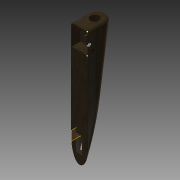
# Autodesk Inventor part: Version 1
Saved by Autodesk Inventor 2015 SP2 (Build 190223200, 223)
## iProperties
Created: 2016-03-30
Part Number: Version 1
Material: Wood (Maple)
Document SubType Name: Modeling
Designer: cvhssub1
Density: 0.67 g/cm^3
Appearance: Natural Maple - Glossy Dark Tint
Author: cvhssub1
Autodesk Inventor part; units mm, degrees
ref_plane "YZ Plane" through (0, 0, 0) normal (1, 0, 0) x (0, 1, 0)
ref_plane "XZ Plane" through (0, 0, 0) normal (0, 1, 0) x (-1, 0, 0)
ref_plane "XY Plane" through (0, 0, 0) normal (0, 0, 1) x (1, 0, 0)
sketch "Sketch2" plane through (0, 0, 0) normal (1, 0, 0) x (0, 1, 0)
  line L0 (0, 0) -> (60, 0)
  line L1 (0, 0) -> (0, -280)
  line L2 (0, -280) -> (20, -280)
  line L3 (20, -280) -> (60, 0)
  dimension "d2" = 60
  dimension "d3" = 280
  dimension "d4" = 20
  constraints: 8 end point, 1 horizontal, 1 perpendicular, 1 vertical
  measures "d2" distance of L0.start L0.end
  measures "d3" distance of L0.start L1.end
  measures "d4" distance of L1.end L2.end
extrude "Extrusion1" add sketch "Sketch2" along normal blind 40
sketch "Sketch3" plane through (0, 0, 0) normal (0, 0, 1) x (1, 0, 0)
  line L0 (0, 35) -> (40, 35)
  line L1 (0, 0) -> (40, 0) projected
  line L2 (0, 60) -> (40, 60) projected
  circle A0 centre (20, 35) radius 10
  dimension "d7" = 35
  dimension "d8" = 20
  dimension "d43" = 35
  constraints: 2 end point, 1 centre point
  measures "d7" distance of L1.start L0.start
  measures "d8" diameter of A0
  measures "d43" distance from line of L1 A0.centre
extrude "Extrusion2" cut sketch "Sketch3" against normal blind 52
fillet "Fillet1" radius 500 1 edges at (20, 20, -280)
full round fillet "Fillet6" first side at (40, 33.1004, -48.2971) centre faces at (13.3333, 53.1004, -48.2971) second side at (0, 33.1004, -48.2971)
fillet "Fillet7" radius 5 5 edges at (40, 19.8985, 0) (0, 19.8985, 0) (5.8578, 54.0827, 0) (20, 60, 0) (34.1422, 54.0827, 0)
fillet "Fillet8" radius 1 8 edges at (38.5355, 0, -1.4645) (40, 0, -115.0253) (20, 0, -280) (36.9375, 0, -256.0741) (3.0625, 0, -256.0741) (0, 0, -115.0253) (1.4645, 0, -1.4645) (20, 0, 0)
sketch "Sketch4" plane through (5, 0, -1) normal (0, -1, 0) x (1, 0, 0)
  line L0 (0, 0) -> (30, 0) projected
  line L1 (34, -4) -> (34, -220.9957) projected
  line L2 (33, -5) -> (33, -47)
  line L3 (33, -47) -> (-3, -47)
  line L4 (-3, -47) -> (-3, -5)
  line L5 (33, -5) -> (-3, -5)
  line L6 (-5, -141.0627) -> (-5, -4) projected
  point P0 (-5, 1)
  dimension "d21" = 42
  dimension "d24" = 5
  constraints: 8 end point, 3 perpendicular, 1 parallel
  measures "d21" distance of L2.start L2.end
  measures "d24" distance between parallel lines of L0 L5
extrude "Extrusion3" cut sketch "Sketch4" against normal blind 20
ref_plane "Work Plane1" through (12, 0, -216.4163) normal (1, 0, 0) x (0, 0, -1)
sketch "Sketch6" plane through (12, 0, -216.4163) normal (1, 0, 0) x (0, 0, -1)
  line L0 (38, 5) -> (0, 5)
  arc A0 (38, 5) -> (0, 5) centre (19, 5) ccw
  line L1 (0, 5) -> (0, -22.1837)
  line L2 (38, 5) -> (38, -22.1837)
  line L3 (38, -22.1837) -> (0, -22.1837)
  point P0 (-216.4163, 0)
  dimension "d38" = 27.1837
  constraints: 8 end point, 3 vertical, 2 point on circle, 2 tangent, 1 centre point, 1 midpoint, 1 perpendicular
  measures "d38" distance from line of L1.end L0
extrude "Extrusion6" cut sketch "Sketch6" along normal blind 14
fillet "Fillet9" radius 1 1 edges at (20, 0, -6)
fillet "Fillet10" radius 1 1 edges at (19, 0, -216.4163)
sketch "Sketch7" plane through (38, 0, -48) normal (-1, 0, 0) x (0, 0, 1)
  line L0 (21, 0) -> (21, 8)
  point P0 (48, 0)
  point P1 (42, 1)
  point P2 (0, 0)
  dimension "d44" = 8
  constraints: 2 end point
  measures "d44" distance of L0.start L0.end
body "Solid1"
